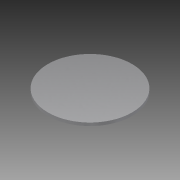
# Autodesk Inventor part: seal1
Saved by Autodesk Inventor 2015 (Build 190159000, 159)
## iProperties
Created: 2015-02-17
Part Number: seal1
Material: Plastic, Transparent
Document SubType Name: Modeling
Designer: Hanjie
Density: 1.188 g/cm^3
Appearance: Transparent - Clear
Mass: 11.5631 g
Surface Area: 82.2133 cm^2
Volume: 9.73322 cm^3
Author: Hanjie
Autodesk Inventor part; units mm, degrees
ref_plane "YZ Plane" through (0, 0, 0) normal (1, 0, 0) x (0, 1, 0)
ref_plane "XZ Plane" through (0, 0, 0) normal (0, 1, 0) x (-1, 0, 0)
ref_plane "XY Plane" through (0, 0, 0) normal (0, 0, 1) x (1, 0, 0)
sketch "Sketch1" plane through (0, 0, 0) normal (0, 1, 0) x (-1, 0, 0)
  circle A0 centre (0, 0) radius 34.925
  dimension "d0" = 69.85
  constraints: 1 centre point, 1 coincident
  measures "d0" diameter of A0
extrude "Extrusion1" add sketch "Sketch1" along normal blind 2.54
body "Solid1"
